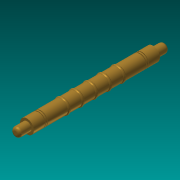
# Autodesk Inventor part: SBM-20
Saved by Autodesk Inventor 2014 SP1 (Build 180222100, 222)
## iProperties
Created: 2014-02-28
Part Number: SBM-20
Material: Brass, Soft Yellow
Document SubType Name: Modeling
Designer: Sawaiz Syed
Density: 8.47 g/cm^3
Appearance: Brass - Satin
Author: Sawaiz Syed
Autodesk Inventor part; units mm, degrees
ref_plane "YZ Plane" through (0, 0, 0) normal (1, 0, 0) x (0, 1, 0)
ref_plane "XZ Plane" through (0, 0, 0) normal (0, 1, 0) x (-1, 0, 0)
ref_plane "XY Plane" through (0, 0, 0) normal (0, 0, 1) x (1, 0, 0)
sketch "Sketch1" plane through (0, 0, 0) normal (0, 0, 1) x (1, 0, 0)
  circle A0 centre (0, 0) radius 5
  dimension "d0" = 10
  constraints: 1 centre point, 1 coincident
  measures "d0" diameter of A0
extrude "Extrusion1" add sketch "Sketch1" along normal mid plane 91
sketch "Sketch2" plane through (0, 0, 45.5) normal (0, 0, 1) x (1, 0, 0)
  circle A0 centre (0, 0) radius 5 projected
  circle A1 centre (0, 0) radius 3.25
  dimension "d3" = 6.5
  constraints: 1 centre point, 1 coincident
  measures "d3" diameter of A1
extrude "Extrusion2" add sketch "Sketch2" along normal blind 8.5 contours A1
sketch "Sketch3" plane through (0, 0, -45.5) normal (0, 0, -1) x (-1, 0, 0)
  circle A0 centre (0, 0) radius 5 projected
  circle A1 centre (0, 0) radius 3.25
  dimension "d6" = 6.5
  constraints: 1 centre point, 1 coincident
  measures "d6" diameter of A1
extrude "Extrusion3" add sketch "Sketch3" along normal blind 8.5 contours A1
fillet "Fillet2" radius 2 1 edges at (3.25, 0, -54)
fillet "Fillet3" radius 2 1 edges at (-3.25, 0, 54)
sketch "Sketch4" plane through (0, 0, 0) normal (0, 0, 1) x (1, 0, 0)
  circle A0 centre (0, 0) radius 5.5
  dimension "d13" = 11
  constraints: 1 centre point, 1 coincident
  measures "d13" diameter of A0
extrude "Extrusion4" add sketch "Sketch4" along normal mid plane 2
pattern_linear "Rectangular Pattern1" count 5 spacing 10 along (0, 0, 1) of "Extrusion4" first direction both ways yes
fillet "Fillet6" radius 1 10 edges at (-5.5, 0, 21) (-5.5, 0, 19) (-5.5, 0, 11) (-5.5, 0, 9) (-5.5, 0, 1) (-5.5, 0, -1) (-5.5, 0, -11) (-5.5, 0, -9) (-5.5, 0, -19) (-5.5, 0, -21)
sketch "Sketch5" plane through (0, 0, 0) normal (1, 0, 0) x (0, 1, 0)
  line L0 (5, 45.5) -> (-5, 45.5) projected
  line L1 (5, 21) -> (-5, 21) projected
  line L2 (5, 37.5) -> (4.5, 37.5)
  line L3 (4.5, 37.5) -> (4.5, 37)
  line L4 (4.5, 37) -> (5, 37)
  line L5 (5, 37) -> (5, 37.5)
  line L6 (5, 36) -> (4.5, 36)
  line L7 (4.5, 36) -> (4.5, 35.5)
  line L8 (4.5, 35.5) -> (5, 35.5)
  line L9 (5, 35.5) -> (5, 36)
  line L10 (5, 45.5) -> (5, 21)
  line L11 (0, 0) -> (15.1316, 0)
  line L12 (5, -45.5) -> (-5, -45.5)
  line L13 (5, -21) -> (-5, -21)
  line L14 (5, -37.5) -> (4.5, -37.5)
  line L15 (4.5, -37.5) -> (4.5, -37)
  line L16 (4.5, -37) -> (5, -37)
  line L17 (5, -37) -> (5, -37.5)
  line L18 (5, -36) -> (4.5, -36)
  line L19 (4.5, -36) -> (4.5, -35.5)
  line L20 (4.5, -35.5) -> (5, -35.5)
  line L21 (5, -35.5) -> (5, -36)
  line L22 (5, -45.5) -> (5, -21)
  line L23 (0, -75.6) -> (0, 75.6) projected
  dimension "d21" = 0.5
  dimension "d22" = 8
  dimension "d23" = 1
  dimension "d24" = 0.5
  dimension "d25" = 0
  dimension "d26" = 0
  dimension "d27" = 0.5
  dimension "d28" = 0.5
  constraints: 42 end point, 12 symmetric about line, 4 parallel, 3 perpendicular, 2 horizontal, 1 collinear
  measures "d21" distance of L2.start L2.end
  measures "d22" distance between parallel lines of L0 L2
  measures "d23" distance between parallel lines of L6 L4
  measures "d24" distance between parallel lines of L7 L9
  measures "d25" distance between parallel lines of L10 L5
  measures "d26" distance between parallel lines of L10 L9
  measures "d27" distance between parallel lines of L8 L6
  measures "d28" distance between parallel lines of L4 L2
revolve "Revolution1" cut sketch "Sketch5" angle 360 about axis through (0, 0, -10) along (0, 0, 1) contours L5 L4 L3 L2 | L9 L8 L7 L6 | L14 L15 L16 L17 | L18 L19 L20 L21
body "Solid1"
